# Autodesk Inventor part: DX3D-SF
Saved by Autodesk Inventor 2013 (Build 170138000, 138)
## iProperties
Created: 2013-01-27
Part Number: DX3D-SF
Material: Generic
Document SubType Name: Modeling
Designer: davidgitz
Density: 1 g/cm^3
Author: davidgitz
Autodesk Inventor part; units mm, degrees
ref_plane "YZ Plane" through (0, 0, 0) normal (1, 0, 0) x (0, 1, 0)
ref_plane "XZ Plane" through (0, 0, 0) normal (0, 1, 0) x (-1, 0, 0)
ref_plane "XY Plane" through (0, 0, 0) normal (0, 0, 1) x (1, 0, 0)
sketch "DM3D-SF, DX3D-SF_53" plane through (0, 0, 0) normal (0, 0, 1) x (1, 0, 0)
  line L0 (-5.8819, 9.2725) -> (7.0721, 9.2725)
  line L1 (7.0721, 9.2725) -> (7.0721, -3.11)
  line L2 (7.0721, -3.11) -> (5.9926, -3.11)
  line L3 (5.9926, -3.11) -> (5.6751, -2.7925)
  line L4 (5.6751, -2.7925) -> (5.6751, -1.205)
  line L5 (5.6751, -1.205) -> (-4.4849, -1.205)
  line L6 (-4.4849, -1.205) -> (-4.4849, -2.7925)
  line L7 (-4.4849, -2.7925) -> (-4.8024, -3.11)
  line L8 (-4.8024, -3.11) -> (-5.8819, -3.11)
  line L9 (-5.8819, -3.11) -> (-5.8819, 9.2725)
  constraints: 20 end point
extrude "Extrusion1" add sketch "DM3D-SF, DX3D-SF_53" along normal blind 6.35
body "Solid1"
